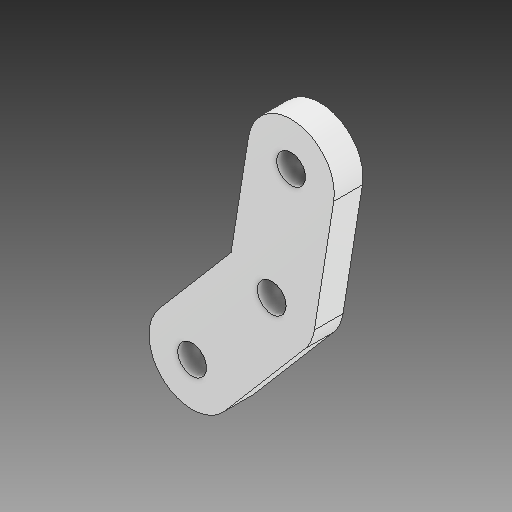
# Autodesk Inventor part: 段ばね抑え2
Saved by Autodesk Inventor 2020 (Build 240168000, 168)
## iProperties
Created: 2019-09-07
Part Number: 段ばね抑え2
Material: アセタール樹脂、白
Document SubType Name: Modeling
Designer: 雪村
Density: 1.425 g/cm^3
Appearance: 滑らか - 白
Mass: 1.16614 g
Surface Area: 8.68694 cm^2
Volume: 0.818345 cm^3
Description: ジュラコン 3t
Author: 雪村
Autodesk Inventor part; units mm, degrees
ref_plane "YZ Plane" through (0, 0, 0) normal (1, 0, 0) x (0, 1, 0)
ref_plane "XZ Plane" through (0, 0, 0) normal (0, 1, 0) x (-1, 0, 0)
ref_plane "XY Plane" through (0, 0, 0) normal (0, 0, 1) x (1, 0, 0)
sketch "スケッチ1" plane through (0, 0, 0) normal (0, 0, 1) x (1, 0, 0)
  circle A0 centre (12.3759, 55.251) radius 1.5
  circle A1 centre (22.7017, 77.6457) radius 1.5
  circle A2 centre (20.6799, 65) radius 1.5
  circle A3 centre (22.7017, 77.6457) radius 4.5
  circle A4 centre (20.6799, 65) radius 4.5
  circle A5 centre (12.3759, 55.251) radius 4.5
  line L0 (8.9502, 58.1689) -> (17.2542, 67.918)
  line L1 (18.2581, 78.3561) -> (16.2364, 65.7104)
  line L2 (27.1453, 76.9352) -> (25.1235, 64.2896)
  line L3 (15.8017, 52.333) -> (24.1057, 62.082)
  point P0 (0, 0)
  point P1 (0, 0)
  point P2 (16.4357, 66.957)
  dimension "d0" = 3
  dimension "d1" = 3
  dimension "d2" = 3
  constraints: 8 end point, 8 point on circle, 8 tangent, 6 centre point, 6 other
  measures "d0" radial gap between concentric circles of A1 A3
  measures "d1" radial gap between concentric circles of A2 A4
  measures "d2" radial gap between concentric circles of A0 A5
extrude "押し出し1" add sketch "スケッチ1" along normal blind 3
